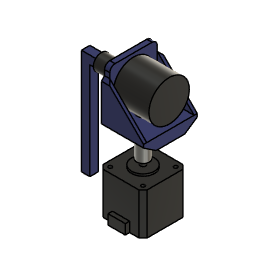
inverted_pendulum_robot_assy (Autodesk Fusion 360 design; units mm, degrees)
Autodesk Fusion 360 part; units mm, degrees
sketch "Sketch1" plane through (0, 0, 0) normal (0, 0, 1) x (1, 0, 0) in component "Stepper Motor"
  line L0 (20.9, 20.9) -> (-20.9, 20.9)
  line L1 (-20.9, 20.9) -> (-20.9, -20.9)
  line L2 (-20.9, -20.9) -> (20.9, -20.9)
  line L3 (20.9, -20.9) -> (20.9, 20.9)
  line L4 (20.9, 20.9) -> (-20.9, -20.9) construction
  line L5 (-20.9, 20.9) -> (20.9, -20.9) construction
  line L6 (-20.9, 17.0009) -> (-17.0009, 20.9)
  line L7 (0, 0) -> (-20.9, 0) construction
  line L8 (-20.9, -17.0009) -> (-17.0009, -20.9)
  line L9 (0, 0) -> (0, 20.9) construction
  line L10 (20.9, 17.0009) -> (17.0009, 20.9)
  line L11 (20.9, -17.0009) -> (17.0009, -20.9)
  line L12 (0, -20.9) -> (0, -22.95) construction
  line L13 (8.2, -20.9) -> (-8.2, -20.9)
  line L14 (-8.2, -20.9) -> (-8.2, -25)
  line L15 (-8.2, -25) -> (8.2, -25)
  line L16 (8.2, -25) -> (8.2, -20.9)
  line L17 (8.2, -20.9) -> (-8.2, -25) construction
  line L18 (-8.2, -20.9) -> (8.2, -25) construction
  point P0 (0, -22.95)
  dimension "d1" = 41.8
  dimension "d2" = 26.8
  dimension "d9" = 16.4
  dimension "d10" = 45.9
  constraint horizontal L0
  constraint perpendicular L0 L1
  constraint parallel L0 L2
  constraint parallel L1 L3
  constraint coincident L4 L7.start
  constraint coincident L5 L7.start
  constraint coincident L7.start L9.start
  constraint equal L0 L3
  constraint coincident L1 L6.start
  constraint coincident L0 L6.end
  constraint parallel L4 L6
  constraint midpoint L1 L7.end
  constraint symmetric L6.start L7 L8.start
  constraint symmetric L6.end L7 L8.end
  constraint midpoint L0 L9.end
  constraint symmetric L6.start L9 L10.start
  constraint symmetric L6.end L9 L10.end
  constraint symmetric L8.start L9 L11.start
  constraint symmetric L8.end L9 L11.end
  constraint midpoint L2 L12.start
  constraint perpendicular L2 L12
  constraint horizontal L13
  constraint perpendicular L13 L14
  constraint parallel L13 L15
  constraint parallel L14 L16
  constraint coincident L17 P0
  constraint coincident L18 P0
  constraint coincident L2 L13.start
  constraint coincident P0 L12.end
  measures "d1" distance of L0.start L0.end
  measures "d2" distance of L7.start L6
  measures "d9" distance of L14 L16
  measures "d10" distance of L0 L15
extrude "Extrude1" add sketch "Sketch1" along normal blind 39.5 contours L0 L1 L2 L3 L6 L8 L10 L11 L13 makes body 1 in component "Stepper Motor"
sketch "Sketch2" plane through (0, 0, 39.5) normal (0, 0, 1) x (-1, 0, 0) in component "Stepper Motor"
  line L0 (-20.9, -17.0009) -> (-17.0009, -20.9)
  line L1 (-17.0009, -20.9) -> (17.0009, -20.9)
  line L2 (17.0009, -20.9) -> (20.9, -17.0009)
  line L3 (20.9, -17.0009) -> (20.9, 17.0009)
  line L4 (20.9, 17.0009) -> (17.0009, 20.9)
  line L5 (17.0009, 20.9) -> (-17.0009, 20.9)
  line L6 (-17.0009, 20.9) -> (-20.9, 17.0009)
  line L7 (-20.9, 17.0009) -> (-20.9, -17.0009)
  circle A0 centre (15.55, -15.55) radius 1.7
  line L8 (15.55, -15.55) -> (15.55, -20.9) construction
  line L9 (15.55, -15.55) -> (20.9, -15.55) construction
  line L10 (20.9, 0) -> (-20.9, 0) construction
  circle A1 centre (15.55, 15.55) radius 1.7
  line L11 (0, 0) -> (0, -20.9) construction
  circle A2 centre (-15.55, -15.55) radius 1.7
  circle A3 centre (-15.55, 15.55) radius 1.7
  circle A4 centre (0, 0) radius 10.9
  circle A5 centre (0, 0) radius 2.5
  dimension "d5" = 5.35
  dimension "d6" = 3.4
  dimension "d13" = 21.8
  dimension "d14" = 5
  constraint coincident A0.centre L8.start
  constraint coincident L1 L8.end
  constraint perpendicular L1 L8
  constraint coincident L3 L9.end
  constraint horizontal L9
  constraint equal L8 L9
  constraint midpoint L3 L10.start
  constraint midpoint L7 L10.end
  constraint symmetric A0 L10 A1
  constraint coincident L11.start A4.centre
  constraint midpoint L1 L11.end
  constraint symmetric A0 L11 A2
  constraint symmetric A1 L11 A3
  measures "d5" distance of A0.centre L8.end
  measures "d6" diameter of A0
  measures "d13" diameter of A4
  measures "d14" diameter of A5
extrude "Extrude2" cut sketch "Sketch2" against normal blind 10 contours A0 | A1 | A2 | A3 bodies 1 in component "Stepper Motor"
extrude "Extrude3" add sketch "Sketch1" along normal blind 9.4 contours L2 L13 L14 L15 L16 bodies 1 in component "Stepper Motor"
extrude "Extrude4" add sketch "Sketch2" along normal blind 1.9 contours A4 bodies 1 in component "Stepper Motor"
extrude "Extrude5" add sketch "Sketch2" along normal blind 22.2 contours A5 bodies 1 in component "Stepper Motor"
sketch "Sketch1 (2)" plane through (0, 0, 0) normal (0, 0, 1) x (1, 0, 0) in component "Rotary Encoder"
  circle A0 centre (0, 0) radius 19.15
  dimension "d19" = 38.3
  constraint coincident A0.centre origin
  measures "d19" diameter of A0
extrude "Extrude1'" add sketch "Sketch1 (2)" along normal blind 33.8 separate body makes body 2 in component "Rotary Encoder"
sketch "Sketch3" plane through (0, 0, 33.8) normal (0, 0, 1) x (-1, 0, 0) in component "Rotary Encoder"
  circle A0 centre (0, 0) radius 19.15
  circle A1 centre (0, 0) radius 9.95
  circle A2 centre (0, 0) radius 7.65
  line L0 (0, 0) -> (-9.447, -16.6576) construction
  circle A3 centre (-7.3751, -13.0042) radius 1.7
  circle A4 centre (-12.0055, -7.1043) radius 1.7
  line L1 (0, 0) -> (-16.4806, -9.7525) construction
  circle A5 centre (12.1022, -6.9383) radius 1.7
  line L2 (0, 0) -> (16.6134, -9.5246) construction
  circle A6 centre (14.95, 0) radius 1.7
  line L3 (0, 0) -> (19.15, 0) construction
  circle A7 centre (-0.4861, 13.9415) radius 1.7
  line L4 (0, 0) -> (-0.6673, 19.1384) construction
  circle A8 centre (-7.3259, 13.032) radius 1.7
  line L5 (0, 0) -> (-9.384, 16.6932) construction
  line L6 (0, 0) -> (-19.15, 0) construction
  dimension "d24" = 19.9
  dimension "d25" = 15.3
  dimension "d31" = 4.2
  dimension "d32" = 3.4
  dimension "d33" = 7.5
  dimension "d34" = 5.2
  dimension "d35" = 20.4
  dimension "d38" = 4.2
  dimension "d39" = 20.8
  dimension "d40" = 5.2
  dimension "d41" = 6.9
  dimension "d42" = 4.2
  dimension "d45" = 7.5
  dimension "d46" = 5.2
  constraint concentric A0 A1
  constraint concentric A1 A2
  constraint coincident A0.centre A1.centre
  constraint coincident A0 L0.end
  constraint coincident L0 A3.centre
  constraint equal A3 A4
  constraint coincident A0 L1.end
  constraint coincident A4.centre L1
  constraint equal A3 A5
  constraint coincident A0 L2.end
  constraint coincident A5.centre L2
  constraint equal A5 A6
  constraint coincident A0 L3.end
  constraint coincident A6.centre L3
  constraint coincident A0 L4.end
  constraint coincident A7.centre L4
  constraint equal A6 A7
  constraint equal A7 A8
  constraint coincident A0 L5.end
  constraint coincident A8.centre L5
  constraint horizontal L3
  constraint coincident A0 L6.end
  constraint horizontal L6
  measures "d24" diameter of A1
  measures "d25" diameter of A2
  measures "d31" distance of L0.end A3.centre
  measures "d32" diameter of A3
  measures "d33" distance of A3.centre A4.centre
  measures "d34" distance of A4.centre L1.end
  measures "d35" distance of A3.centre A5.centre
  measures "d38" distance of A6.centre L3.end
  measures "d39" distance of A6.centre A7.centre
  measures "d40" distance of A7.centre L4.end
  measures "d41" distance of A7.centre A8.centre
  measures "d42" distance of A8.centre L5.end
  measures "d45" distance of A5.centre A6.centre
  measures "d46" distance of A5.centre L2.end
extrude "Extrude3'" add sketch "Sketch3" along normal blind 30.5 contours A2 bodies 2 in component "Rotary Encoder"
extrude "Extrude2'" add sketch "Sketch3" along normal blind 5 contours A1 | A2 bodies 2 in component "Rotary Encoder"
sketch "Sketch4" plane through (0, 0, 64.3) normal (0, 0, 1) x (-1, 0, 0) in component "Rotary Encoder"
  circle A0 centre (0, 0) radius 7.65
  circle A1 centre (0, 0) radius 2.9
  dimension "d28" = 5.8
  constraint concentric A0 A1
  measures "d28" diameter of A1
extrude "Extrude4'" cut sketch "Sketch4" against normal blind 6 contours A1 bodies 2 in component "Rotary Encoder"
extrude "Extrude5'" cut sketch "Sketch3" against normal blind 5 contours A3 | A4 | A5 | A6 | A7 | A8 bodies 2 in component "Rotary Encoder"
sketch "Sketch1 (3)" plane through (0, 0, 145.2773) normal (0, 0, 1) x (-1, 0, 0) in component "Encoder Housing"
  circle A0 centre (14.4589, -13.9264) radius 1.7
  circle A1 centre (21.3479, 13.0194) radius 1.7
  circle A2 centre (33.9362, -7.8604) radius 1.7
  circle A3 centre (9.8286, -8.0264) radius 1.7
  circle A4 centre (14.5081, 12.1099) radius 1.7
  circle A5 centre (36.784, -0.9221) radius 1.7
  circle A6 centre (21.834, -0.9221) radius 9.95
  circle A7 centre (21.834, -0.9221) radius 19.15
  line L0 (-0.666, 21.5779) -> (44.334, 21.5779)
  line L1 (44.334, 21.5779) -> (44.334, -23.4221)
  line L2 (44.334, -23.4221) -> (-0.666, -23.4221)
  line L3 (-0.666, -23.4221) -> (-0.666, 21.5779)
  line L4 (-0.666, 21.5779) -> (44.334, -23.4221) construction
  line L5 (44.334, 21.5779) -> (-0.666, -23.4221) construction
  circle A8 centre (21.834, -0.9221) radius 10.35
  circle A9 centre (21.834, -0.9221) radius 9.95
  point P0 (21.834, -0.9221)
  dimension "d47" = 45
  dimension "d50" = 0.4
  constraint horizontal L0
  constraint perpendicular L0 L1
  constraint parallel L0 L2
  constraint parallel L1 L3
  constraint coincident L4 P0
  constraint coincident L5 P0
  constraint coincident P0 A6.centre
  constraint equal L0 L3
  measures "d47" distance of L0.start L0.end
  measures "d50" distance of A8 A9
extrude "Extrude1''" add sketch "Sketch1 (3)" along normal blind 5 separate body contours A1 | A2 | A3 | A7 | L0 L1 L2 L3 makes body 3 in component "Encoder Housing"
cylinder "CylinderPrimitive1" add diameter 11.9 height 25.3 placed x (1, 0, 0) y (0, 1, 0) z (0, 0, 1) at (0, 0, 0) separate body makes body 4 in component "Motor Coupler"
sketch "Sketch3 (2)" plane through (0, 0, 25.3) normal (0, 0, 1) x (-1, 0, 0) in component "Motor Coupler"
  circle A0 centre (0, 0) radius 5.95
  circle A1 centre (0, 0) radius 3.05
  dimension "d57" = 6.1
  constraint concentric A0 A1
  measures "d57" diameter of A1
extrude "Extrude1'''" cut sketch "Sketch3 (2)" against normal blind 25.3 contours A1 bodies 4 in component "Motor Coupler"
sketch "Sketch2 (2)" plane through (-44.334, 0, 0) normal (-1, 0, 0) x (0, -1, 0) in component "Encoder Housing"
  line L0 (-23.4221, 145.2773) -> (21.5779, 145.2773)
  line L1 (21.5779, 145.2773) -> (21.5779, 150.2773)
  line L2 (21.5779, 150.2773) -> (-23.4221, 150.2773)
  line L3 (-23.4221, 150.2773) -> (-23.4221, 145.2773)
  line L4 (-23.4221, 150.2773) -> (21.5779, 150.2773)
  line L5 (21.5779, 150.2773) -> (21.5779, 110.2773)
  line L6 (21.5779, 110.2773) -> (-23.4221, 110.2773)
  line L7 (-23.4221, 110.2773) -> (-23.4221, 150.2773)
  line L8 (-0.9221, 110.2773) -> (-0.9221, 150.2773) construction
  circle A0 centre (-0.9221, 136.2773) radius 3.2
  line L9 (-0.9221, 130.2773) -> (-23.4221, 130.2773) construction
  circle A1 centre (-0.9221, 136.2773) radius 5.3
  line L10 (-23.4221, 150.2773) -> (-26.4221, 150.2773)
  line L11 (-26.4221, 150.2773) -> (-26.4221, 110.2773)
  line L12 (-26.4221, 110.2773) -> (-23.4221, 110.2773)
  line L13 (-23.4221, 110.2773) -> (-23.4221, 150.2773)
  line L14 (21.5779, 150.2773) -> (24.5779, 150.2773)
  line L15 (24.5779, 150.2773) -> (24.5779, 110.2773)
  line L16 (24.5779, 110.2773) -> (21.5779, 110.2773)
  line L17 (21.5779, 110.2773) -> (21.5779, 150.2773)
  dimension "d64" = 40
  dimension "d65" = 6.4
  dimension "d66" = 6
  dimension "d67" = 10.6
  dimension "d78" = 3
  constraint horizontal L4
  constraint vertical L5
  constraint horizontal L6
  constraint vertical L7
  constraint coincident L2.end L3.start
  constraint collinear L1 L5
  constraint midpoint L6 L8.start
  constraint midpoint L4 L8.end
  constraint coincident L8 A0.centre
  constraint midpoint L8 L9.start
  constraint midpoint L7 L9.end
  constraint concentric A0 A1
  constraint horizontal L10
  constraint vertical L11
  constraint horizontal L12
  constraint vertical L13
  constraint collinear L6 L12
  constraint horizontal L14
  constraint vertical L15
  constraint horizontal L16
  constraint vertical L17
  constraint collinear L6 L16
  constraint equal L10 L14
  measures "d64" distance of L1.end L5.end
  measures "d65" diameter of A0
  measures "d66" distance of A0.centre L9.start
  measures "d67" diameter of A1
  measures "d78" distance of L2.end L10.end
extrude "Extrude2''" add sketch "Sketch2 (2)" along normal blind 11 separate body contours L0 L1 L2 L3 L4 L5 L7 L13 L17 | L0 L5 L6 L7 L13 L17 | A1 makes body 5 in component "Encoder Housing"
extrude "Extrude3''" cut sketch "Sketch2 (2)" along normal blind 4 contours A1 bodies 5 in component "Encoder Housing"
extrude "Extrude4''" add sketch "Sketch2 (2)" along normal blind 11 and the other way blind 35 contours L3 L7 L10 L11 L12 L13 | L1 L5 L14 L15 L16 L17 bodies 3 5 in component "Encoder Housing"
chamfer "Chamfer1" distance 35 angle 45 2 edges at (-9.334, 24.9221, 110.2773) (-9.334, -23.0779, 110.2773) on bodies 3 in component "Encoder Housing"
fillet "Fillet2" radius 5 2 edges at (0.666, 23.4221, 147.7773) (0.666, -21.5779, 147.7773) on bodies 3 in component "Encoder Housing"
chamfer "Chamfer2" distance 3 angle 45 2 edges at (-9.334, -24.5779, 147.7773) (-9.334, 26.4221, 147.7773) on bodies 3 in component "Encoder Housing"
chamfer "Chamfer3" distance 12 distance2 8 2 edges at (-55.334, 26.4221, 130.2773) (-55.334, -24.5779, 130.2773) measured on face at (-55.334, 1.0018, 117.8803) measured on face at (-55.334, 1.0018, 117.8803) on bodies 3 in component "Encoder Housing"
sketch "Sketch1 (4)" plane through (0, 0, 145.2773) normal (0, 0, 1) x (-1, 0, 0) in component "Encoder Housing (1)"
  circle A0 centre (14.4589, -13.9264) radius 1.7
  circle A1 centre (21.3479, 13.0194) radius 1.7
  circle A2 centre (33.9362, -7.8604) radius 1.7
  circle A3 centre (9.8286, -8.0264) radius 1.7
  circle A4 centre (14.5081, 12.1099) radius 1.7
  circle A5 centre (36.784, -0.9221) radius 1.7
  circle A6 centre (20.834, -0.9221) radius 9.95
  circle A7 centre (20.834, -0.9221) radius 19.15
  line L0 (-1.666, 21.5779) -> (43.334, 21.5779)
  line L1 (43.334, 21.5779) -> (43.334, -23.4221)
  line L2 (43.334, -23.4221) -> (-1.666, -23.4221)
  line L3 (-1.666, -23.4221) -> (-1.666, 21.5779)
  line L4 (-1.666, 21.5779) -> (43.334, -23.4221) construction
  line L5 (43.334, 21.5779) -> (-1.666, -23.4221) construction
  circle A8 centre (20.834, -0.9221) radius 9.95
  circle A9 centre (20.834, -0.9221) radius 9.55
  circle A10 centre (14.4589, -13.9264) radius 1.7
  circle A11 centre (21.3479, 13.0194) radius 1.7
  circle A12 centre (33.9362, -7.8604) radius 1.7
  circle A13 centre (9.8286, -8.0264) radius 1.7
  circle A14 centre (14.5081, 12.1099) radius 1.7
  circle A15 centre (36.784, -0.9221) radius 1.7
  circle A16 centre (21.834, -0.9221) radius 9.95
  circle A17 centre (21.834, -0.9221) radius 19.15
  circle A18 centre (20.834, -0.9221) radius 9.95
  point P0 (20.834, -0.9221)
  point P1 (20.834, -0.9221)
  dimension "d47_1" = 45
  dimension "d50_1" = 0.4
  constraint horizontal L0
  constraint perpendicular L0 L1
  constraint parallel L0 L2
  constraint parallel L1 L3
  constraint coincident L4 P1
  constraint coincident L5 P1
  constraint coincident P1 P0
  constraint equal L0 L3
  constraint equal A7 A17
  constraint equal A6 A8
  constraint equal A8 A18
  measures "d47_1" distance of L0.start L0.end
  measures "d50_1" distance of A8 A9
extrude "Extrude1''''" add sketch "Sketch1 (4)" along normal blind 5 separate body contours A1 A11 | A2 A12 | A3 A13 | A6 A8 A16 A18 | A7 A17 | A7 A17 | A7 A17 | L0 L1 L2 L3 makes body 6 in component "Encoder Housing (1)"
sketch "Sketch2 (3)" plane through (-43.334, 0, 0) normal (-1, 0, 0) x (0, -1, 0) in component "Encoder Housing (1)"
  line L0 (-23.4221, 145.2773) -> (21.5779, 145.2773)
  line L1 (21.5779, 145.2773) -> (21.5779, 150.2773)
  line L2 (21.5779, 150.2773) -> (-23.4221, 150.2773)
  line L3 (-23.4221, 150.2773) -> (-23.4221, 145.2773)
  line L4 (-23.4221, 150.2773) -> (21.5779, 150.2773)
  line L5 (21.5779, 150.2773) -> (21.5779, 110.2773)
  line L6 (21.5779, 110.2773) -> (-23.4221, 110.2773)
  line L7 (-23.4221, 110.2773) -> (-23.4221, 150.2773)
  line L8 (-0.9221, 110.2773) -> (-0.9221, 150.2773) construction
  circle A0 centre (-0.9221, 136.2773) radius 3.2
  line L9 (-0.9221, 130.2773) -> (-23.4221, 130.2773) construction
  circle A1 centre (-0.9221, 136.2773) radius 5.3
  line L10 (-23.4221, 150.2773) -> (-26.4221, 150.2773)
  line L11 (-26.4221, 150.2773) -> (-26.4221, 110.2773)
  line L12 (-26.4221, 110.2773) -> (-23.4221, 110.2773)
  line L13 (-23.4221, 110.2773) -> (-23.4221, 150.2773)
  line L14 (21.5779, 150.2773) -> (24.5779, 150.2773)
  line L15 (24.5779, 150.2773) -> (24.5779, 110.2773)
  line L16 (24.5779, 110.2773) -> (21.5779, 110.2773)
  line L17 (21.5779, 110.2773) -> (21.5779, 150.2773)
  dimension "d64_1" = 40
  dimension "d65_1" = 6.4
  dimension "d66_1" = 6
  dimension "d67_1" = 10.6
  dimension "d78_1" = 3
  constraint horizontal L4
  constraint vertical L5
  constraint horizontal L6
  constraint vertical L7
  constraint coincident L2.end L3.start
  constraint collinear L1 L5
  constraint midpoint L6 L8.start
  constraint midpoint L4 L8.end
  constraint coincident L8 A0.centre
  constraint midpoint L8 L9.start
  constraint midpoint L7 L9.end
  constraint concentric A0 A1
  constraint horizontal L10
  constraint vertical L11
  constraint horizontal L12
  constraint vertical L13
  constraint collinear L6 L12
  constraint horizontal L14
  constraint vertical L15
  constraint horizontal L16
  constraint vertical L17
  constraint collinear L6 L16
  constraint equal L10 L14
  measures "d64_1" distance of L1.end L5.end
  measures "d65_1" diameter of A0
  measures "d66_1" distance of A0.centre L9.start
  measures "d67_1" diameter of A1
  measures "d78_1" distance of L2.end L10.end
extrude "Extrude2'''" add sketch "Sketch2 (3)" along normal blind 12 separate body contours L0 L1 L2 L3 L4 L5 L7 L13 L17 | L0 L5 L6 L7 L13 L17 | A1 makes body 7 in component "Encoder Housing (1)"
extrude "Extrude3'''" cut sketch "Sketch2 (3)" along normal blind 6 contours A1 bodies 7 in component "Encoder Housing (1)"
extrude "Extrude4'''" add sketch "Sketch2 (3)" along normal blind 12 and the other way blind 35 contours L3 L7 L10 L11 L12 L13 | L1 L5 L14 L15 L16 L17 bodies 6 7 in component "Encoder Housing (1)"
chamfer "Chamfer1'" distance 35 angle 45 2 edges at (-8.334, 24.9221, 110.2773) (-8.334, -23.0779, 110.2773) on bodies 6 in component "Encoder Housing (1)"
fillet "Fillet2'" radius 5 2 edges at (1.666, 23.4221, 147.7773) (1.666, -21.5779, 147.7773) on bodies 6 in component "Encoder Housing (1)"
chamfer "Chamfer2'" distance 3 angle 45 2 edges at (-8.334, -24.5779, 147.7773) (-8.334, 26.4221, 147.7773) on bodies 6 in component "Encoder Housing (1)"
chamfer "Chamfer3'" distance 12 distance2 8 2 edges at (-55.334, 26.4221, 130.2773) (-55.334, -24.5779, 130.2773) measured on face at (-55.334, 0.8424, 117.8803) measured on face at (-55.334, 0.8424, 117.8803) on bodies 6 in component "Encoder Housing (1)"
sketch "Sketch3 (3)" plane through (-55.334, 0, 0) normal (-1, 0, 0) x (0, -1, 0) in component "Encoder Housing (1)"
  line L0 (12.5779, 150.2773) -> (-14.4221, 150.2773)
  line L1 (-14.4221, 110.2773) -> (12.5779, 110.2773)
  circle A0 centre (-0.9221, 136.2773) radius 3.2
  line L2 (-5.0221, 128.2773) -> (3.1779, 128.2773)
  line L3 (3.1779, 128.2773) -> (3.1779, 144.2773)
  line L4 (3.1779, 144.2773) -> (-5.0221, 144.2773)
  line L5 (-5.0221, 144.2773) -> (-5.0221, 128.2773)
  line L6 (-5.0221, 128.2773) -> (3.1779, 144.2773) construction
  line L7 (3.1779, 128.2773) -> (-5.0221, 144.2773) construction
  line L8 (12.5779, 110.2773) -> (12.5779, 150.2773)
  line L9 (-14.4221, 150.2773) -> (-14.4221, 110.2773)
  point P0 (-0.9221, 136.2773)
  dimension "d94" = 16
  dimension "d95" = 8.2
  constraint horizontal L2
  constraint perpendicular L2 L3
  constraint parallel L2 L4
  constraint parallel L3 L5
  constraint coincident L6 P0
  constraint coincident L7 P0
  constraint coincident P0 A0.centre
  measures "d94" distance of L2.start L4.end
  measures "d95" distance of L3.end L4.end
extrude "Extrude5''" cut sketch "Sketch3 (3)" against normal blind 3 contours L2 L3 L4 L5 bodies 6 in component "Encoder Housing (1)"
sketch "Sketch1 (5)" plane through (0, 0, 0) normal (1, 0, 0) x (0, 1, 0) in component "Pendulum"
  line L0 (0, 0) -> (25, 0)
  line L1 (25, 0) -> (25, 4.6)
  line L2 (25, 4.6) -> (0, 4.6)
  line L3 (0, 4.6) -> (0, 0)
  line L4 (25, 4.6) -> (17, 4.6)
  line L5 (17, 4.6) -> (17, -93.7)
  line L6 (17, -93.7) -> (25, -93.7)
  line L7 (25, -93.7) -> (25, 4.6)
  line L8 (25, 6.3) -> (10, 6.3)
  line L9 (10, 6.3) -> (10, -1.7)
  line L10 (10, -1.7) -> (25, -1.7)
  line L11 (25, -1.7) -> (25, 6.3)
  line L12 (25, 6.3) -> (10, -1.7) construction
  line L13 (10, 6.3) -> (25, -1.7) construction
  line L14 (0, 2.3) -> (25, 2.3) construction
  point P0 (17.5, 2.3)
  dimension "d98" = 4.6
  dimension "d99" = 8
  dimension "d100" = 10
  dimension "d101" = 8
  dimension "d102" = 25
  dimension "d103" = 100
  constraint horizontal L0
  constraint vertical L1
  constraint horizontal L2
  constraint vertical L3
  constraint coincident L0.start L3.end
  constraint horizontal L4
  constraint vertical L5
  constraint horizontal L6
  constraint vertical L7
  constraint horizontal L8
  constraint perpendicular L8 L9
  constraint parallel L8 L10
  constraint parallel L9 L11
  constraint coincident L12 P0
  constraint coincident L13 P0
  constraint midpoint L12 P0
  constraint collinear L7 L11
  constraint midpoint L3 L14.start
  constraint midpoint L11 L14.end
  constraint coincident P0 L14
  measures "d98" distance of L0.start L2.end
  measures "d99" distance of L8.end L9.end
  measures "d100" distance of L3 L9
  measures "d101" distance of L5.end L6.end
  measures "d102" distance of L14.start L14.end
  measures "d103" distance of L6.end L8.start
extrude "Extrude1'''''" add sketch "Sketch1 (5)" along normal mid plane 4.6 separate body contours L0 L2 L3 L9 makes body 8 in component "Pendulum"
extrude "Extrude2''''" add sketch "Sketch1 (5)" along normal mid plane 8 contours L0 L2 L5 L9 | L0 L5 L9 L10 | L0 L1 L2 L4 L5 L7 L11 | L0 L5 L7 L10 L11 | L2 L4 L8 L9 L11 | L5 L6 L7 L10 bodies 8 in component "Pendulum"
fillet "Fillet1" radius 2.3 4 edges at (2.3, 5, 4.6) (2.3, 5, 0) (-2.3, 5, 4.6) (-2.3, 5, 0) on bodies 8 in component "Pendulum"
sketch "Sketch3 (4)" plane through (0, 0, -93.7) normal (0, 0, -1) x (1, 0, 0) in component "Pendulum"
  line L0 (-4, -25) -> (4, -25)
  line L1 (4, -25) -> (4, -17)
  line L2 (4, -17) -> (-4, -17)
  line L3 (-4, -17) -> (-4, -25)
  line L4 (-4, -17) -> (4, -25) construction
  line L5 (-4, -25) -> (4, -17) construction
  line L6 (0, -18.4019) -> (-2.25, -19.701)
  line L7 (-2.25, -19.701) -> (-2.25, -22.299)
  line L8 (-2.25, -22.299) -> (0, -23.5981)
  line L9 (0, -23.5981) -> (2.25, -22.299)
  line L10 (2.25, -22.299) -> (2.25, -19.701)
  line L11 (2.25, -19.701) -> (0, -18.4019)
  line L12 (0, -21) -> (0, -18.4019) construction
  point P0 (0, -21)
  point P1 (0, -21)
  dimension "d126" = 4.5
  constraint coincident L2.end L3.start
  constraint coincident L0.end L1.start
  constraint coincident L0.start L3.end
  constraint coincident L1.end L2.start
  constraint coincident L5 P1
  constraint coincident L4 P1
  constraint coincident P1 P0
  constraint vertical L12
  measures "d126" distance of L7 L10
sketch "Sketch2 (4)" plane through (0, 0, 0) normal (0, -1, 0) x (1, 0, 0) in component "Pendulum"
  line L0 (-1.5969, 4.1) -> (1.5969, 4.1)
  line L1 (0, 4.1) -> (0, 4.6) construction
  circle A0 centre (0, 2.3) radius 2.3
  dimension "d128" = 0.5
  constraint horizontal L0
  constraint midpoint L0 L1.start
  constraint perpendicular L0 L1
  constraint coincident L1.end A0
  measures "d128" distance of L1.start L1.end
extrude "Extrude4''''" cut sketch "Sketch2 (4)" against normal blind 10 contours L0 A0 picked at (-0.1703, 4.2475) bodies 8 in component "Pendulum"
sketch "Sketch1 (6)" plane through (0, 0, 0) normal (1, 0, 0) x (0, 1, 0) in component "Pendulum (1)"
  line L0 (0, 0) -> (25, 0)
  line L1 (25, 0) -> (25, 4.6)
  line L2 (25, 4.6) -> (0, 4.6)
  line L3 (0, 4.6) -> (0, 0)
  line L4 (25, 4.6) -> (17, 4.6)
  line L5 (17, 4.6) -> (17, -63.7)
  line L6 (17, -63.7) -> (25, -63.7)
  line L7 (25, -63.7) -> (25, 4.6)
  line L8 (25, 6.3) -> (10, 6.3)
  line L9 (10, 6.3) -> (10, -1.7)
  line L10 (10, -1.7) -> (25, -1.7)
  line L11 (25, -1.7) -> (25, 6.3)
  line L12 (25, 6.3) -> (10, -1.7) construction
  line L13 (10, 6.3) -> (25, -1.7) construction
  line L14 (0, 2.3) -> (25, 2.3) construction
  point P0 (17.5, 2.3)
  dimension "d98_1" = 4.6
  dimension "d99_1" = 8
  dimension "d100_1" = 10
  dimension "d101_1" = 8
  dimension "d102_1" = 25
  dimension "d103_1" = 70
  constraint horizontal L0
  constraint vertical L1
  constraint horizontal L2
  constraint vertical L3
  constraint coincident L0.start L3.end
  constraint horizontal L4
  constraint vertical L5
  constraint horizontal L6
  constraint vertical L7
  constraint horizontal L8
  constraint perpendicular L8 L9
  constraint parallel L8 L10
  constraint parallel L9 L11
  constraint coincident L12 P0
  constraint coincident L13 P0
  constraint midpoint L12 P0
  constraint collinear L7 L11
  constraint midpoint L3 L14.start
  constraint midpoint L11 L14.end
  constraint coincident P0 L14
  measures "d98_1" distance of L0.start L2.end
  measures "d99_1" distance of L8.end L9.end
  measures "d100_1" distance of L3 L9
  measures "d101_1" distance of L5.end L6.end
  measures "d102_1" distance of L14.start L14.end
  measures "d103_1" distance of L6.end L8.start
extrude "Extrude1''''''" add sketch "Sketch1 (6)" along normal mid plane 4.6 separate body contours L0 L2 L3 L9 makes body 9 in component "Pendulum (1)"
extrude "Extrude2'''''" add sketch "Sketch1 (6)" along normal mid plane 8 contours L0 L2 L5 L9 | L0 L5 L9 L10 | L0 L1 L2 L4 L5 L7 L11 | L0 L5 L7 L10 L11 | L2 L4 L8 L9 L11 | L5 L6 L7 L10 bodies 9 in component "Pendulum (1)"
fillet "Fillet1'" radius 2.3 4 edges at (2.3, 5, 4.6) (2.3, 5, 0) (-2.3, 5, 4.6) (-2.3, 5, 0) on bodies 9 in component "Pendulum (1)"
sketch "Sketch3 (5)" plane through (0, 0, -63.7) normal (0, 0, -1) x (1, 0, 0) in component "Pendulum (1)"
  line L0 (-4, -25) -> (4, -25)
  line L1 (4, -25) -> (4, -17)
  line L2 (4, -17) -> (-4, -17)
  line L3 (-4, -17) -> (-4, -25)
  line L4 (-4, -17) -> (4, -25) construction
  line L5 (-4, -25) -> (4, -17) construction
  line L6 (0, -18.4019) -> (-2.25, -19.701)
  line L7 (-2.25, -19.701) -> (-2.25, -22.299)
  line L8 (-2.25, -22.299) -> (0, -23.5981)
  line L9 (0, -23.5981) -> (2.25, -22.299)
  line L10 (2.25, -22.299) -> (2.25, -19.701)
  line L11 (2.25, -19.701) -> (0, -18.4019)
  line L12 (0, -21) -> (0, -18.4019) construction
  point P0 (0, -21)
  point P1 (0, -21)
  dimension "d126_1" = 4.5
  constraint coincident L2.end L3.start
  constraint coincident L0.end L1.start
  constraint coincident L0.start L3.end
  constraint coincident L1.end L2.start
  constraint coincident L5 P1
  constraint coincident L4 P1
  constraint coincident P1 P0
  constraint vertical L12
  measures "d126_1" distance of L7 L10
extrude "Extrude3''''" add sketch "Sketch3 (5)" along normal blind 18 contours L6 L7 L8 L9 L10 L11 bodies 9 in component "Pendulum (1)"
sketch "Sketch2 (5)" plane through (0, 0, 0) normal (0, -1, 0) x (1, 0, 0) in component "Pendulum (1)"
  line L0 (-1.5969, 4.1) -> (1.5969, 4.1)
  line L1 (0, 4.1) -> (0, 4.6) construction
  circle A0 centre (0, 2.3) radius 2.3
  dimension "d128_1" = 0.5
  constraint horizontal L0
  constraint midpoint L0 L1.start
  constraint perpendicular L0 L1
  constraint coincident L1.end A0
  measures "d128_1" distance of L1.start L1.end
extrude "Extrude4'''''" cut sketch "Sketch2 (5)" against normal blind 10 contours L0 A0 picked at (-0.1703, 4.2475) bodies 9 in component "Pendulum (1)"
chamfer "Chamfer1''" distance 0.5 angle 45 6 edges at (1.125, 19.0514, -81.7) (2.25, 21, -81.7) (1.125, 22.9486, -81.7) (-1.125, 22.9486, -81.7) (-2.25, 21, -81.7) (-1.125, 19.0514, -81.7) on bodies 9 in component "Pendulum (1)"
chamfer "Chamfer4" [suppressed] in component "Encoder Housing (1)"
sketch "Sketch3 (6)" plane through (-55.334, 0, 0) normal (-1, 0, 0) x (0, -1, 0) in component "Encoder Housing"
  line L0 (12.5779, 110.2773) -> (12.5779, 150.2773)
  line L1 (12.5779, 150.2773) -> (-14.4221, 150.2773)
  line L2 (-14.4221, 150.2773) -> (-14.4221, 110.2773)
  line L3 (-14.4221, 110.2773) -> (12.5779, 110.2773)
  circle A0 centre (-0.9221, 136.2773) radius 3.2
  line L4 (-5.0221, 128.2773) -> (3.1779, 128.2773)
  line L5 (3.1779, 128.2773) -> (3.1779, 144.2773)
  line L6 (3.1779, 144.2773) -> (-5.0221, 144.2773)
  line L7 (-5.0221, 144.2773) -> (-5.0221, 128.2773)
  line L8 (-5.0221, 128.2773) -> (3.1779, 144.2773) construction
  line L9 (3.1779, 128.2773) -> (-5.0221, 144.2773) construction
  point P0 (-0.9221, 136.2773)
  dimension "d121" = 16
  dimension "d122" = 8.2
  constraint horizontal L4
  constraint perpendicular L4 L5
  constraint parallel L4 L6
  constraint parallel L5 L7
  constraint coincident L8 P0
  constraint coincident L9 P0
  constraint coincident P0 A0.centre
  measures "d121" distance of L4.start L6.end
  measures "d122" distance of L4.start L4.end
extrude "Extrude5'''" [suppressed] in component "Encoder Housing"
chamfer "Chamfer4'" [suppressed] in component "Encoder Housing"
component "Stepper Motor" placed x (1, 0, 0) y (0, 1, 0) z (0, 0, 1) at (0, 0, 0)
component "Rotary Encoder" placed x (0, 0, 1) y (0, 1, 0) z (-1, 0, 0) at (24.8, 0, 106.2)
component "Motor Coupler" placed x (1, 0, 0) y (0, 1, 0) z (0, 0, 1) at (0, 0, 46.4)
component "Pendulum" placed x (0, 1, 0) y (-1, 0, 0) z (0, 0, 1) at (-29.5, 0, 103.9)
component "Encoder Housing" placed x (0, 0, 1) y (0, 1, 0) z (-1, 0, 0) at (136.2773, -0.9221, 128.034)
component "Encoder Housing" placed x (0, 0, 1) y (0, 1, 0) z (-1, 0, 0) at (136.2773, -0.9221, 128.034)
equation "d2 = ( 53.6 / 2 ) * 1 mm"
equation "d5 = 4 mm + ( 2.7 / 2 ) * 1 mm"
equation "d26 = 64.30 mm - 33.8 mm"
equation "d31 = 2.85 mm + ( 2.7 / 2 ) * 1 mm"
equation "d33 = 4.8 mm + 2.7 mm"
equation "d34 = 3.85 mm + ( 2.7 / 2 ) * 1 mm"
equation "d35 = 17.4 mm + 3 mm"
equation "d39 = 17.8 mm + 3 mm"
equation "d41 = 4.2 mm + 2.7 * 1 mm"
equation "d68 = 6 mm + 5 mm"
equation "d68_1 = 6 mm + 6 mm"
